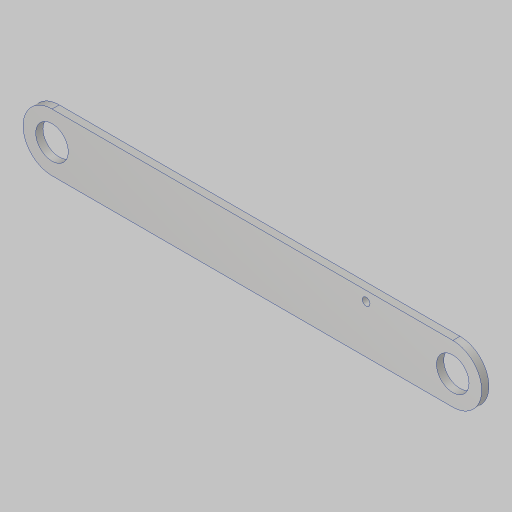
# Autodesk Inventor part: GP4-002
Saved by Autodesk Inventor 2023.5 (Build 275446000, 446)
## iProperties
Created: 2025-02-23
Part Number: GP4-002
Material: Aluminum 6061
Document SubType Name: Modeling
Designer: slick
Density: 2.7 g/cm^3
Appearance: Aluminum - Flat
Author: slick
Autodesk Inventor part; units mm, degrees
ref_plane "YZ Plane" through (0, 0, 0) normal (1, 0, 0) x (0, 1, 0)
ref_plane "XZ Plane" through (0, 0, 0) normal (0, 1, 0) x (-1, 0, 0)
ref_plane "XY Plane" through (0, 0, 0) normal (0, 0, 1) x (1, 0, 0)
sketch "Sketch1" plane through (0, 0, 0) normal (0, 0, 1) x (1, 0, 0)
  circle A0 centre (0, 0) radius 14.2875
  circle A1 centre (352.3742, 0) radius 14.2875
  line L0 (0, 0) -> (352.3742, 0) construction
  line L1 (0, 0) -> (352.3742, 0) construction
  line L2 (0, -25.4) -> (352.3742, -25.4)
  line L3 (352.3742, 25.4) -> (0, 25.4)
  arc A2 (0, 25.4) -> (0, -25.4) centre (0, 0) ccw
  arc A3 (352.3742, -25.4) -> (352.3742, 25.4) centre (352.3742, 0) ccw
  point P0 (176.1871, 0)
  dimension "d0" = 28.575
  dimension "d1" = 352.3742
  dimension "d2" = 50.8
  constraints: 10 end point, 4 centre point, 4 point on circle, 4 tangent, 2 equal length, 1 coincident, 1 equal radius, 1 horizontal, 1 midpoint
  measures "d0" diameter of A0
  measures "d1" distance of L0.start L0.end
  measures "d2" diameter of A3
extrude "Extrusion1" add sketch "Sketch1" along normal blind 6.35
sketch "Sketch2" plane through (0, 0, 6.35) normal (0, 0, 1) x (1, 0, 0)
  circle A0 centre (0, 0) radius 14.2875 construction
  circle A1 centre (0, 0) radius 14.2875 construction
  circle A2 centre (352.3742, 0) radius 14.2875 construction
  line L0 (0, 0) -> (352.3742, 0) construction
  line L1 (276.225, 16.8402) -> (276.225, 0) construction
  dimension "d14" = 276.225
  dimension "d15" = 16.8402
  constraints: 4 end point, 1 horizontal, 1 perpendicular, 1 point on line
  measures "d14" distance of L1.end point (0, 0)
  measures "d15" distance from line of L0 L1.start
hole "Hole1" at (276.225, 16.8402, 6.35) direction (0, 0, -1) diameter 6.7564 end through all clearance for "Flat Head Machine Screw (82)" size "1/4" standard "Ansi Unified Screw Threads"
body "Solid1"
